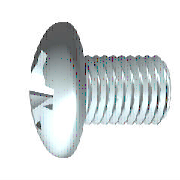
# Autodesk Inventor part: ANSI B18.6.3 - 0 - 80 - 3/16
Saved by Autodesk Inventor 2013 (Build 170138000, 138)
## iProperties
IsCustomPart: 0
Created: 2010-02-08
Part Number: ANSI B18.6.3 - 0 - 80 - 3/16
Material: Steel, Mild
Description: Cross Recessed Pan Head Machine Screw - Type IA
Document SubType Name: Modeling
Standard: ANSI B18.6.3
Designer: Phillip
Standard Revision: 2003
Standards Organization: ANSI
Language: en-US
Size Designation: 0 - 80 - 3/16
Categories: <MemberInstance><Categories><Category DisplayName="Fasteners" InternalName="e4da775c-781d-43d5-af7c-5136215cf5a6" Mnemonic="FSTN"><Category DisplayName="Bolts" InternalName="536e6df0-f778-49ac-b2f2-25c71d2aa0b2" Mnemonic="SCRW"><CategoryParameter DisplayName="Nominal Diameter" InternalName="8bbe3f8e-44cf-40a9-a251-3a6edc8168d6" Mnemonic="nomdia"/><CategoryParameter DisplayName="Nominal Length" InternalName="238ecbaf-3e6c-45dd-aa95-4068c8e0fd02" Mnemonic="nomlen"/><CategoryParameter DisplayName="Thread Series Designation" InternalName="87c5849c-b3a5-4c3e-9c9b-2feecef9be86" Mnemonic="thrserdsgn"/><CategoryParameter DisplayName="Thread Class" InternalName="ebc0d23b-2cc6-4d2a-b376-d52aae53bab6" Mnemonic="thrclss"/><CategoryParameter DisplayName="Thread Designation" InternalName="586d5e89-370a-4089-914f-0110033585c7" Mnemonic="thrdesign"/><CategoryParameter DisplayName="Thread Type" InternalName="b4bbb7bc-d6aa-4c9f-a9a9-4152b9f6fe49" Mnemonic="thrtype"/><CategoryParameter DisplayName="Threads per Unit" InternalName="bdc6e7d2-ffd0-4d9c-a173-16b95ebb912d" Mnemonic="thrperunit1"/><CategoryParameter DisplayName="Thread Pitch" InternalName="bb82302e-82d8-4176-8fc1-c5d7bb17d5ad" Mnemonic="pitch1"/><CategoryParameter DisplayName="Nominal Diameter Designation" InternalName="03caf894-eafd-4c09-a035-916ac084b87b" Mnemonic="nomdiadesig"/><Category DisplayName="Round Head" InternalName="df3578aa-538f-4805-96a8-2439eb0c3cf7" Mnemonic="RNDSCRW"><CategoryParameter DisplayName="Shank Diameter" InternalName="c22f1a48-b8d5-43ef-ac5e-546ba91c0bd6" Mnemonic="grpdia"/><CategoryParameter DisplayName="Grip Length" InternalName="2c6ace26-543b-4217-91c4-9cdf8c3ec6f1" Mnemonic="grplen"/><CategoryParameter DisplayName="Thread Length" InternalName="a1e5edc5-4ca7-4847-8786-65b14d35af16" Mnemonic="thrlen"/><CategoryParameter DisplayName="Head Diameter" InternalName="e71ee7a1-06fd-425c-ba3b-09769885677c" Mnemonic="headdia"/><CategoryParameter DisplayName="Head Height" InternalName="2d152238-84fe-49ae-94c3-3fee884c292b" Mnemonic="headh"/><CategoryParameter DisplayName="Property Class" InternalName="85496db6-1567-48ed-b0d4-aa1f03366005" Mnemonic="propclss"/></Category></Category></Category><Category DisplayName="DataType" InternalName="23b78d0f-2648-40c6-8793-ca6db495c9e8" Mnemonic="DATATYPE"><CategoryParameter DisplayName="DisplayName" InternalName="05415f3d-3907-474b-a020-eb9d644f4cf3" Mnemonic="DISPLAYNAME"/><CategoryParameter DisplayName="InternalName" InternalName="cf1d0246-76d9-4b4a-8305-fa0409afb5c1" Mnemonic="INTERNALNAME"/><CategoryParameter DisplayName="Folder Name" InternalName="3f06958e-8713-4116-9be7-ed6184ecc97b" Mnemonic="FOLDERNAME"/><CategoryParameter DisplayName="Family Version" InternalName="914462f6-6e19-4b14-ba84-155b9680b1d0" Mnemonic="FAMILYREVISION"/><CategoryParameter DisplayName="ClipFormat" InternalName="bc51e27b-3422-4e78-93ef-cec197ddf230" Mnemonic="CLIPFORMAT"/><CategoryParameter DisplayName="IsMetric" InternalName="e2385c5b-1ea4-4823-96a8-8de651266ec3" Mnemonic="ISMETRIC"/><CategoryParameter DisplayName="Description" InternalName="13903e3d-64b1-4950-80da-f627842ea37f" Mnemonic="DESCRIPTION"/><CategoryParameter DisplayName="StdsOrg" InternalName="8f5914e1-4693-403f-8ab5-d37768198c9d" Mnemonic="STDSORG"/><CategoryParameter DisplayName="Standard" InternalName="0c0a119c-1e12-4c84-803f-101930972f5e" Mnemonic="STANDARD"/><CategoryParameter DisplayName="Manufacturer" InternalName="cd6c7a72-a28a-4e50-99a9-2c7f4e13e5ad" Mnemonic="MANUFACTURER"/><CategoryParameter DisplayName="Member Revision" InternalName="a65d44b9-392f-4f4f-857b-e4b3d54996fe" Mnemonic="MEMBERREVISION"/><CategoryParameter DisplayName="Standard Revision" InternalName="91d5a463-65c2-4fde-b823-3b7fea5e8e17" Mnemonic="STANDARDREVISION"/><CategoryParameter DisplayName="Revision Guid" InternalName="45a75005-10b1-4dfc-8d6d-dfe629f0b93c" Mnemonic="REVISIONGUID"/><CategoryParameter DisplayName="Designation" InternalName="2675968c-4ce5-49e0-a4f5-552d29089031" Mnemonic="DESIGNATION"/><CategoryParameter DisplayName="FileName" InternalName="8b46a4cc-9585-4fed-90c3-899f57e09a73" Mnemonic="FILENAME"/><CategoryParameter DisplayName="Default Row" InternalName="2af9ec52-faaa-4026-b378-f9fa4afca842" Mnemonic="DEFAULTROW"/><Category DisplayName="Part" InternalName="c0e0b642-3bcb-4cc8-9e80-f96d35c4afa4" Mnemonic="PART"><CategoryParameter DisplayName="Material" InternalName="818a152a-d3c3-49ca-80ee-df7d91421b8e" Mnemonic="MATERIAL"/><CategoryParameter DisplayName="Material Key" InternalName="5c9a8adb-dd2b-4535-b97f-0a94a95fe41f" Mnemonic="MATERIALKEY"/><CategoryParameter DisplayName="Part Number" InternalName="016b6077-bfbe-49bd-92c9-d8d59c39c941" Mnemonic="PARTNUMBER"/><CategoryParameter DisplayName="Stock Number" InternalName="4dba7c1c-e26c-444e-836c-b08b433409a8" Mnemonic="STOCKNUMBER"/></Category></Category><Category DisplayName="Legacy Map DA" InternalName="924fff40-ddd0-4eff-ad42-30e3774ef79e" Mnemonic="LEGACYMAPDA"><CategoryParameter DisplayName="DACookie" InternalName="316934ee-8fe1-4c7a-9c36-f2d79e1add1a" Mnemonic="DACOOKIE"/></Category><Category DisplayName="LegacyMap" InternalName="cd87c42b-3e48-431e-b5c0-1cbeb14dfe77" Mnemonic="LEGACYMAP"><CategoryParameter DisplayName="CatalogName" InternalName="d99d1e27-aa94-4de2-af4c-c348882a6f4f" Mnemonic="CATALOGNAME"/><CategoryParameter DisplayName="FamilyNumber" InternalName="e705e1f4-09cb-413e-91f9-551b4188271e" Mnemonic="FAMILYNUMBER"/><CategoryParameter DisplayName="MemberID" InternalName="8e5e0294-fc51-4c8f-b3d7-003dc5ed94f6" Mnemonic="MEMBERID"/><CategoryParameter DisplayName="unique CC member ID" InternalName="5193edd4-b2b0-4ab4-9d54-de900eee34e0" Mnemonic="CCCOOKIE"/><CategoryParameter DisplayName="unique DA member ID" InternalName="0918ad47-427f-4fed-ae26-24c81c58f590" Mnemonic="DACOOKIE"/><CategoryParameter DisplayName="Merge11 ID" InternalName="0ee8fb18-e2ed-4f39-96f6-1f4b5f50aa71" Mnemonic="MERGE11"/><CategoryParameter DisplayName="Split ID" InternalName="72b5c83c-be7f-45c4-ae51-9160ea6deb26" Mnemonic="SPLIT"/></Category></Categories><FamilyTemplate Id="si0152"><FamilyTemplateParameters><FamilyTemplateParameter ObjectType="kUserParameterObject" ValueType="xs:double" Id="1" ObjectReferenceKey="GUL"/><FamilyTemplateParameter ObjectType="kUserParameterObject" ValueType="xs:double" Id="2" ObjectReferenceKey="SPD"/><FamilyTemplateParameter ObjectType="kUserParameterObject" ValueType="xs:double" Id="3" ObjectReferenceKey="NLG"/><FamilyTemplateParameter ObjectType="kUserParameterObject" ValueType="xs:double" Id="4" ObjectReferenceKey="KOD"/><FamilyTemplateParameter ObjectType="kUserParameterObject" ValueType="xs:double" Id="5" ObjectReferenceKey="SBR"/><FamilyTemplateParameter ObjectType="kUserParameterObject" ValueType="xs:double" Id="6" ObjectReferenceKey="KR"/><FamilyTemplateParameter ObjectType="kUserParameterObject" ValueType="xs:double" Id="7" ObjectReferenceKey="PTC"/><FamilyTemplateParameter ObjectType="kUserParameterObject" ValueType="xs:double" Id="8" ObjectReferenceKey="GEL"/><FamilyTemplateParameter ObjectType="kUserParameterObject" ValueType="xs:double" Id="9" ObjectReferenceKey="THREADDIA"/><FamilyTemplateParameter ObjectType="kUserParameterObject" ValueType="xs:double" Id="10" ObjectReferenceKey="TOA"/><FamilyTemplateParameter ObjectType="kUserParameterObject" ValueType="xs:double" Id="11" ObjectReferenceKey="BDM"/><FamilyTemplateParameter ObjectType="kUserParameterObject" ValueType="xs:double" Id="12" ObjectReferenceKey="RR"/><FamilyTemplateParameter ObjectType="kUserParameterObject" ValueType="xs:double" Id="13" ObjectReferenceKey="STI"/><FamilyTemplateParameter ObjectType="kUserParameterObject" ValueType="xs:double" Id="14" ObjectReferenceKey="TPU"/><FamilyTemplateParameter ObjectType="kUserParameterObject" ValueType="xs:double" Id="15" ObjectReferenceKey="KOH"/><FamilyTemplateParameter ObjectType="kUserParameterObject" ValueType="xs:double" Id="16" ObjectReferenceKey="SDM"/><FamilyTemplateParameter ObjectType="kUserParameterObject" ValueType="xs:double" Id="17" ObjectReferenceKey="NND"/><FamilyTemplateParameter ObjectType="kUserParameterObject" ValueType="xs:double" Id="18" ObjectReferenceKey="GD"/><FamilyTemplateParameter ObjectType="kUserParameterObject" ValueType="xs:double" Id="19" ObjectReferenceKey="GAL"/><FamilyTemplateParameter ObjectType="kUserParameterObject" ValueType="xs:double" Id="20" ObjectReferenceKey="KEWI"/><FamilyTemplateParameter ObjectType="kUserParameterObject" ValueType="xs:double" Id="21" ObjectReferenceKey="GD1"/><FamilyTemplateParameter ObjectType="kPropertyObject" ValueType="xs:string" Id="100" ObjectReferenceKey="{32853F0F-3444-11d1-9E93-0060B03C1CA6}" SubObjectId="52"/><FamilyTemplateParameter ObjectType="kPropertyObject" ValueType="xs:string" Id="105" ObjectReferenceKey="{32853F0F-3444-11d1-9E93-0060B03C1CA6}" SubObjectId="5"/><FamilyTemplateParameter ObjectType="kPartComponentDefinitionObject" ValueType="xs:string" Id="110" SubObjectId="Material"/><FamilyTemplateParameter ObjectType="kThreadFeatureObject" ValueType="xs:structure" Id="300" ObjectReferenceKey="1002000010000000aa0f0000000000008000000000000000" SubObjectId="ThreadInfo"><FamilyTemplateParameter ObjectType="" ValueType="xs:string" Id="301" SubObjectId="ThreadDesignation"/><FamilyTemplateParameter ObjectType="" ValueType="xs:string" Id="302" SubObjectId="ThreadType"/><FamilyTemplateParameter ObjectType="" ValueType="xs:string" Id="303" SubObjectId="ThreadClass"/></FamilyTemplateParameter></FamilyTemplateParameters></FamilyTemplate><CategoryParameterMap><ParamToTemplateMap><ParamToTemplate CategoryParameter="//CategoryParameter[@InternalName='05415f3d-3907-474b-a020-eb9d644f4cf3']" ConstantValue="Cross Recessed Pan Head Machine Screw - Type IA - Inch"/><ParamToTemplate CategoryParameter="//CategoryParameter[@InternalName='cf1d0246-76d9-4b4a-8305-fa0409afb5c1']" ConstantValue="cfb9df52-93fc-4fcb-a3a5-3466ef0e77aa"/><ParamToTemplate CategoryParameter="//CategoryParameter[@InternalName='3f06958e-8713-4116-9be7-ed6184ecc97b']" ConstantValue="ANSI B18.6.3(25)"/><ParamToTemplate CategoryParameter="//CategoryParameter[@InternalName='914462f6-6e19-4b14-ba84-155b9680b1d0']" ConstantValue="10"/><ParamToTemplate CategoryParameter="//CategoryParameter[@InternalName='bc51e27b-3422-4e78-93ef-cec197ddf230']" ConstantValue="CF_INVENTOR.STDPARTS"/><ParamToTemplate CategoryParameter="//CategoryParameter[@InternalName='e2385c5b-1ea4-4823-96a8-8de651266ec3']" ConstantValue="false"/><ParamToTemplate CategoryParameter="//CategoryParameter[@InternalName='13903e3d-64b1-4950-80da-f627842ea37f']" ConstantValue="Cross Recessed Pan Head Machine Screw - Type IA"/><ParamToTemplate CategoryParameter="//CategoryParameter[@InternalName='8f5914e1-4693-403f-8ab5-d37768198c9d']" ConstantValue="ANSI"/><ParamToTemplate CategoryParameter="//CategoryParameter[@InternalName='0c0a119c-1e12-4c84-803f-101930972f5e']" ConstantValue="ANSI B18.6.3"/><ParamToTemplate CategoryParameter="//CategoryParameter[@InternalName='cd6c7a72-a28a-4e50-99a9-2c7f4e13e5ad']" TemplateParameter="104"/><ParamToTemplate CategoryParameter="//CategoryParameter[@InternalName='91d5a463-65c2-4fde-b823-3b7fea5e8e17']" ConstantValue="2003"/><ParamToTemplate CategoryParameter="//CategoryParameter[@InternalName='45a75005-10b1-4dfc-8d6d-dfe629f0b93c']" ConstantValue="12b63537-317b-4092-b5a6-85084c208d10"/><ParamToTemplate CategoryParameter="//CategoryParameter[@InternalName='2af9ec52-faaa-4026-b378-f9fa4afca842']" ConstantValue="10"/><ParamToTemplate CategoryParameter="//CategoryParameter[@InternalName='d99d1e27-aa94-4de2-af4c-c348882a6f4f']" ConstantValue="ANSI"/><ParamToTemplate CategoryParameter="//CategoryParameter[@InternalName='8b46a4cc-9585-4fed-90c3-899f57e09a73']" ConstantValue="ANSI B18.6.3 - 0-80 UNF - 0.1875(5)"/><ParamToTemplate CategoryParameter="//CategoryParameter[@InternalName='a65d44b9-392f-4f4f-857b-e4b3d54996fe']" ConstantValue="1099ce10-b5e3-4895-8f28-d9c0c888e786"/><ParamToTemplate CategoryParameter="//CategoryParameter[@InternalName='2c6ace26-543b-4217-91c4-9cdf8c3ec6f1']" ConstantValue="0.03125"/><ParamToTemplate CategoryParameter="//CategoryParameter[@InternalName='ebc0d23b-2cc6-4d2a-b376-d52aae53bab6']" ConstantValue="2A"/><ParamToTemplate CategoryParameter="//CategoryParameter[@InternalName='87c5849c-b3a5-4c3e-9c9b-2feecef9be86']" ConstantValue="UNF"/><ParamToTemplate CategoryParameter="//CategoryParameter[@InternalName='03caf894-eafd-4c09-a035-916ac084b87b']" ConstantValue="#0"/><ParamToTemplate CategoryParameter="//CategoryParameter[@InternalName='b4bbb7bc-d6aa-4c9f-a9a9-4152b9f6fe49']" ConstantValue="ANSI Unified Screw Threads"/><ParamToTemplate CategoryParameter="//CategoryParameter[@InternalName='e705e1f4-09cb-413e-91f9-551b4188271e']" ConstantValue=""/><ParamToTemplate CategoryParameter="//CategoryParameter[@InternalName='8e5e0294-fc51-4c8f-b3d7-003dc5ed94f6']" ConstantValue=""/><ParamToTemplate CategoryParameter="//CategoryParameter[@InternalName='316934ee-8fe1-4c7a-9c36-f2d79e1add1a']" ConstantValue="*Ans~A1863I2~0-80x0.1875~0.1875~UNF*"/><ParamToTemplate CategoryParameter="//CategoryParameter[@InternalName='c22f1a48-b8d5-43ef-ac5e-546ba91c0bd6']" TemplateParameter="11"/><ParamToTemplate CategoryParameter="//CategoryParameter[@InternalName='2675968c-4ce5-49e0-a4f5-552d29089031']" TemplateParameter="100"/><ParamToTemplate CategoryParameter="//CategoryParameter[@InternalName='a1e5edc5-4ca7-4847-8786-65b14d35af16']" TemplateParameter="8"/><ParamToTemplate CategoryParameter="//CategoryParameter[@InternalName='e71ee7a1-06fd-425c-ba3b-09769885677c']" TemplateParameter="4"/><ParamToTemplate CategoryParameter="//CategoryParameter[@InternalName='2d152238-84fe-49ae-94c3-3fee884c292b']" TemplateParameter="15"/><ParamToTemplate CategoryParameter="//CategoryParameter[@InternalName='818a152a-d3c3-49ca-80ee-df7d91421b8e']" TemplateParameter="110"/><ParamToTemplate CategoryParameter="//CategoryParameter[@InternalName='238ecbaf-3e6c-45dd-aa95-4068c8e0fd02']" TemplateParameter="3"/><ParamToTemplate CategoryParameter="//CategoryParameter[@InternalName='8bbe3f8e-44cf-40a9-a251-3a6edc8168d6']" TemplateParameter="17"/><ParamToTemplate CategoryParameter="//CategoryParameter[@InternalName='016b6077-bfbe-49bd-92c9-d8d59c39c941']" TemplateParameter="105"/><ParamToTemplate CategoryParameter="//CategoryParameter[@InternalName='bb82302e-82d8-4176-8fc1-c5d7bb17d5ad']" TemplateParameter="7"/><ParamToTemplate CategoryParameter="//CategoryParameter[@InternalName='586d5e89-370a-4089-914f-0110033585c7']" TemplateParameter="301"/><ParamToTemplate CategoryParameter="//CategoryParameter[@InternalName='bdc6e7d2-ffd0-4d9c-a173-16b95ebb912d']" TemplateParameter="14"/></ParamToTemplateMap></CategoryParameterMap></MemberInstance>
Density: 1 g/cm^3
Author: Phillip
Autodesk Inventor part; units mm, degrees
ref_plane "YZ Plane" through (0, 0, 0) normal (1, 0, 0) x (0, 1, 0)
sketch "Sketch1" plane through (0, 0, 0) normal (0, 0, 1) x (1, 0, 0)
  line L0 (4.7625, 0) -> (4.7625, 0.762)
  line L1 (4.7625, 0.762) -> (0.79375, 0.762)
  line L2 (3.9624, 5.08) -> (3.9624, 5.08)
  arc A0 (-0.426172, 1.4732) -> (-1.1176, 0) centre (0.79756, 0) ccw
  line L3 (-1.1176, 0) -> (-1.1176, 1.4732)
  line L4 (-0.955873, 0.770266) -> (-0.350735, 0.468555)
  line L5 (-0.350735, 0.468555) -> (-0.1016, 0)
  line L6 (-0.1016, 0) -> (4.7625, 0)
  line L7 (-2.490733, 0) -> (5.971372, 0)
  line L8 (0, -1.016) -> (0, 6.096)
  line L9 (-0.955873, 0.770266) -> (-1.1176, 0.8509) construction
  line L10 (-0.426172, 1.4732) -> (-1.1176, 1.4732)
  line L11 (-0.426172, 1.4732) -> (0, 1.4732)
  line L12 (0, 1.4732) -> (0, 0.762)
  line L13 (0, 0.762) -> (0.47625, 0.762)
  line L14 (0.47625, 0.762) -> (0.79375, 0.762)
  line L15 (0.79375, 0.762) -> (0, 0.762) construction
  dimension "d1" = 1.524
  dimension "d2" = 1.016
  dimension "d16" = 1.7018
  dimension "d17" = 62
  dimension "d19" = 26.5
  dimension "d23" = 2.9464
  dimension "d24" = 0
  dimension "d25" = 1.1176
  dimension "d26" = 1.91516
  dimension "d28" = 1.524
  dimension "d29" = 3.96875
  dimension "d30" = 0.3175
  dimension "d31" = 4.7625
  constraints: 28 end point, 5 collinear, 5 point on line, 4 point on circle, 2 parallel, 2 perpendicular, 1 centre point, 1 horizontal, 1 tangent
  measures "d1" diameter of L1 L6
  measures "d2" distance from line of L5.end L3
  measures "d16" diameter of L9.end L6
  measures "d17" angle of L5 L6
  measures "d19" angle of L4 L6
  measures "d23" diameter of L11.end L6
  measures "d24" angle of L11 L6
  measures "d25" distance between parallel lines of L3 L12
  measures "d26" radius of A0
  measures "d28" diameter of L13 L6
  measures "d29" distance of L0.end L1.end
  measures "d30" distance of L13.end L1.end
  measures "d31" distance between parallel lines of L12 L0
revolve "Body" add sketch "Sketch1" angle 360 about axis through (-0.1016, 0, 0) along (1, 0, 0) contours L6 L8 L13 L14 L1 L0 | L6 L5 L4 A0 L11 L8
ref_plane "Work Plane1" through (-1.1176, 0, 0) normal (1, 0, 0) x (0, 1, 0)
sketch "Sketch2" plane through (-1.1176, 0, 0) normal (1, 0, 0) x (0, 1, 0)
  circle A0 centre (0, 0) radius 1.4732
  line L0 (-3.111971, 0) -> (8.359425, 0)
  line L1 (0, -3.111971) -> (0, 8.359425)
  line L2 (0, 0.8509) -> (0, 0) construction
  line L3 (0, 0) -> (0.8509, 0) construction
  arc A1 (0.34036, 0) -> (0, 0.34036) centre (0, 0) ccw construction
  line L4 (0, 0) -> (6.720654, 6.720654) construction
  line L5 (0.2286, 0.819618) -> (0.129261, 0.405339)
  line L6 (0.819618, 0.2286) -> (0.405339, 0.129261)
  arc A2 (0.129261, 0.405339) -> (0.306251, 0.306251) centre (0.231736, 0.380766) ccw
  arc A3 (0.306251, 0.306251) -> (0.405339, 0.129261) centre (0.380766, 0.231736) ccw
  arc A4 (0.8509, 0) -> (0.819618, 0.2286) centre (0, 0) ccw
  arc A5 (0.2286, 0.819618) -> (0, 0.8509) centre (0, 0) ccw
  arc A6 (0.819618, 0.2286) -> (0.2286, 0.819618) centre (0, 0) ccw
  line L7 (0.2286, -0.819618) -> (0.129261, -0.405339)
  line L8 (0.819618, -0.2286) -> (0.405339, -0.129261)
  arc A7 (0.306251, -0.306251) -> (0.129261, -0.405339) centre (0.231736, -0.380766) ccw
  arc A8 (0.405339, -0.129261) -> (0.306251, -0.306251) centre (0.380766, -0.231736) ccw
  arc A9 (0.819618, -0.2286) -> (0.8509, 0) centre (0, 0) ccw
  arc A10 (0, -0.8509) -> (0.2286, -0.819618) centre (0, 0) ccw
  arc A11 (0.2286, -0.819618) -> (0.819618, -0.2286) centre (0, 0) ccw
  line L9 (-0.2286, 0.819618) -> (-0.129261, 0.405339)
  line L10 (-0.819618, 0.2286) -> (-0.405339, 0.129261)
  arc A12 (-0.306251, 0.306251) -> (-0.129261, 0.405339) centre (-0.231736, 0.380766) ccw
  arc A13 (-0.405339, 0.129261) -> (-0.306251, 0.306251) centre (-0.380766, 0.231736) ccw
  arc A14 (-0.819618, 0.2286) -> (-0.8509, 0) centre (0, 0) ccw
  arc A15 (0, 0.8509) -> (-0.2286, 0.819618) centre (0, 0) ccw
  arc A16 (-0.2286, 0.819618) -> (-0.819618, 0.2286) centre (0, 0) ccw
  arc A17 (-0.2286, -0.819618) -> (0, -0.8509) centre (0, 0) ccw
  arc A18 (-0.819618, -0.2286) -> (-0.2286, -0.819618) centre (0, 0) ccw
  arc A19 (-0.8509, 0) -> (-0.819618, -0.2286) centre (0, 0) ccw
  line L11 (-0.819618, -0.2286) -> (-0.405339, -0.129261)
  line L12 (-0.2286, -0.819618) -> (-0.129261, -0.405339)
  arc A20 (-0.129261, -0.405339) -> (-0.306251, -0.306251) centre (-0.231736, -0.380766) ccw
  arc A21 (-0.306251, -0.306251) -> (-0.405339, -0.129261) centre (-0.380766, -0.231736) ccw
  arc A22 (0.42545, 0) -> (0, 0.42545) centre (0, 0) ccw construction
  dimension "d4" = 45
  dimension "d5" = 0.68072
  dimension "d6" = 1.7018
  dimension "d7" = 0.2286
  dimension "d20" = 0.8509
  constraints: 46 point on circle, 25 symmetric about line, 22 centre point, 22 end point, 6 tangent, 4 coincident, 3 collinear, 3 point on line, 1 midpoint, 1 perpendicular, 22 other
  measures "d4" angle of L4 L3
  measures "d5" diameter of A1
  measures "d6" diameter of A6
  measures "d7" distance from line of L5.start L2
  measures "d20" diameter of A22
extrude "Slot" add sketch "Sketch2" along normal up to next draft 5 contours L6 A3 A2 L5 A6 | A11 L7 A7 A8 L8 | L9 A12 A13 L10 A16 | A18 L11 A21 A20 L12
revolve "Cut" cut sketch "Sketch1" angle 360 about axis through (-10, 0, 0) along (1, 0, 0) contours L3 L10 A0
sketch "Sketch4" plane through (-1.1176, 0, 0) normal (1, 0, 0) x (0, 1, 0)
  circle A0 centre (0, 0) radius 1.4732
  line L0 (-8.99977, 0) -> (8.99977, 0)
  line L1 (0, -8.99977) -> (0, 8.99977)
  line L2 (0, 0) -> (6.428407, 6.428407) construction
  circle A1 centre (0, 0) radius 0.1143 construction
  line L3 (0, 0) -> (6.428407, -6.428407) construction
  line L4 (0, 0) -> (-6.428407, 6.428407) construction
  line L5 (0, 0) -> (-6.428407, -6.428407) construction
  line L6 (0.601677, 0.601677) -> (0, 0.1143)
  line L7 (-0.601677, 0.601677) -> (-0.1143, 0)
  line L8 (-0.601677, -0.601677) -> (0, -0.1143)
  line L9 (0.601677, -0.601677) -> (0.1143, 0)
  line L10 (0.601677, 0.601677) -> (0.1143, 0)
  line L11 (-0.601677, 0.601677) -> (0, 0.1143)
  line L12 (-0.601677, -0.601677) -> (-0.1143, 0)
  line L13 (0.601677, -0.601677) -> (0, -0.1143)
  circle A2 centre (0, 0) radius 0.8509 construction
  dimension "d11" = 0.2286
  dimension "d14" = 45
  dimension "d35" = 0.60168
  constraints: 24 end point, 10 point on line, 7 point on circle, 3 perpendicular, 3 symmetric about line, 2 centre point, 2 coincident, 3 other
  measures "d11" diameter of A1
  measures "d14" angle of L2 L0
  measures "d35" distance from line of L0 L6.start
extrude "Star Cut" cut sketch "Sketch4" along normal blind 1.1176 draft -10 contours L9 L13 L1 L0 | L0 L1 L6 L10 | L1 L0 L7 L11 | L8 L12 L0 L1
fillet "Fillet1" radius 0.383032 1 edges at (-0.4262, -1.4732, 0)
fillet "Fillet2" radius 0.09144 5 edges at (-0.9559, 0, 0.7703) (-0.9559, -0.7703, 0) (-0.9559, 0, -0.7703) (-0.9559, 0.7639, 0.0989) (-0.9559, 0.7639, -0.0989)
thread "Thread" size "0-80 UNF" class "2A" standard "ANSI Unified Screw Threads" length 3.9688
chamfer "Chamfer1" distance 0.15875 distance2 0.0001 1 edges at (4.7625, -0.762, 0) measured on face at (4.7625, 0.1466, 0.4667)
ref_plane "Work Plane3" through (1.85, 0, 0) normal (0, 1, 0) x (1, 0, 0)
equation "\"d11\" = 0.5 * SBR"
equation "\"d35\" = 0.353553 * SDM"
equation "\"d12\" = KOH"
equation "\"d5\" = 0.4 * SDM"
equation "\"d6\" = SDM"
equation "\"d7\" = 0.5 * SBR"
equation "\"d20\" = 0.5 * SDM"
equation "\"d1\" = GD"
equation "\"d2\" = STI"
equation "\"d16\" = SDM"
equation "\"d23\" = KOD"
equation "\"d25\" = KOH"
equation "\"d26\" = KR"
equation "\"d28\" = BDM"
equation "\"d29\" = GEL"
equation "\"d30\" = GAL"
equation "\"d31\" = NLG"
equation "\"d32\" = RR"
equation "\"d22\" = 0.2 * SBR"
equation "\"d8\" = GEL"
equation "\"d36\" = -0.5 * SPD + 0.5 * GD"
equation "\"GD\" = NND"
equation "\"NLG\" = 4.7625"
equation "\"GEL\" = 3.96875"
equation "\"KOD\" = 2.9464"
equation "\"KOH\" = 1.1176"
equation "\"SDM\" = 1.7018"
equation "\"STI\" = 1.016"
equation "\"SBR\" = 0.4572"
equation "\"KEWI\" = 0"
equation "\"d3\" = -KOH"
equation "\"KR\" = 0.65 * KOD"
equation "\"BDM\" = NND"
equation "\"GAL\" = 0.3175"
equation "\"GUL\" = 0"
equation "\"RR\" = 0.13 * KOD"
equation "\"SPD\" = 1.2065"
equation "\"THREADDIA\" = 1.524"
equation "\"TOA\" = 30deg"
equation "\"NND\" = 1.524"
equation "\"GD1\" = 1.2065"
body "Solid1"
